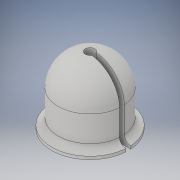
# Autodesk Inventor part: Puller
Saved by Autodesk Inventor 2019 (Build 230136000, 136)
## iProperties
Created: 2018-06-09
Part Number: Puller
Material: Generic
Document SubType Name: Modeling
Designer: kaich
Density: 1 g/cm^3
Appearance: Default
Author: kaich
Autodesk Inventor part; units mm, degrees
ref_plane "YZ Plane" through (0, 0, 0) normal (1, 0, 0) x (0, 1, 0)
ref_plane "XZ Plane" through (0, 0, 0) normal (0, 1, 0) x (-1, 0, 0)
ref_plane "XY Plane" through (0, 0, 0) normal (0, 0, 1) x (1, 0, 0)
sketch "Sketch1" plane through (0, 0, 0) normal (0, 0, 1) x (1, 0, 0)
  arc A0 (0, 4.9998) -> (-5, -0.0002) centre (0, -0.0002) ccw
  arc A1 (-6, -5.028) -> (-5, -4.028) centre (-6, -4.028) ccw
  line L0 (0, -5.5) -> (-6, -5.5)
  line L1 (-6, -5.5) -> (-6, -5.028)
  line L2 (-5, -0.0002) -> (-5, -4.028)
  arc A2 (0, 3.4998) -> (-3.5, -0.0002) centre (0, -0.0002) ccw
  line L3 (-3.5, -0.0002) -> (-3.5, -5.5)
  line L4 (0, 4.9998) -> (0, -5.5)
  point P0 (0, 0)
  dimension "d7" = 90
  dimension "d9" = 6
  dimension "d13" = 1
  dimension "d16" = 10.4998
  dimension "d17" = 5
  dimension "d18" = 3.5
  dimension "d19" = 90
  dimension "d21" = 5.5
  dimension "d22" = 5
  dimension "d23" = 3.5
  constraints: 10 end point, 7 point on circle, 3 centre point, 3 point on line, 3 tangent, 2 perpendicular, 1 coincident, 1 horizontal, 1 vertical
  measures "d9" distance of L0.start L0.end
  measures "d13" distance of A1.end A1.centre
  measures "d16" distance from line of L4.start L0
  measures "d17" radius of A0
  measures "d18" radius of A2
  measures "d19" angle of L4 L0
  measures "d21" distance from line of point (0, 0) L0
  measures "d22" distance from line of A1.end L4
  measures "d23" distance from line of point (0, 0) L3
revolve "Revolution1" add sketch "Sketch1" angle 360 about axis through (0, 4.9998, 0) along (0, -1, 0) contours L4 A2 L3 L0 L1 A1 L2 A0
sketch "Sketch2" plane through (0, 0, 0) normal (0, 1, 0) x (-1, 0, 0)
  point P0 (0, 0)
sketch "Sketch3" plane through (0, 0, 0) normal (0, 1, 0) x (-1, 0, 0)
  circle A0 centre (0, 0) radius 0.75
  dimension "d25" = 1.5
  constraints: 1 centre point, 1 coincident
  measures "d25" diameter of A0
extrude "Extrusion1" cut sketch "Sketch3" along normal up to surface
sketch "Sketch4" plane through (0, 0, 0) normal (1, 0, 0) x (0, 1, 0)
  line L0 (-5.5, -6) -> (-5.5, 6) projected
  line L1 (5.5, -0.375) -> (-5.5, -0.375)
  line L2 (-5.5, -0.375) -> (-5.5, 0.375)
  line L3 (-5.5, 0.375) -> (5.5, 0.375)
  line L4 (5.5, 0.375) -> (5.5, -0.375)
  line L5 (5.5, -0.375) -> (-5.5, 0.375) construction
  line L6 (-5.5, -0.375) -> (5.5, 0.375) construction
  point P0 (0, 0)
  dimension "d28" = 0.75
  constraints: 12 end point, 2 midpoint, 2 parallel, 1 horizontal, 1 perpendicular, 1 point on line
  measures "d28" distance of L3.end L1.start
extrude "Extrusion2" cut sketch "Sketch4" along normal up to surface
body "Solid1"
